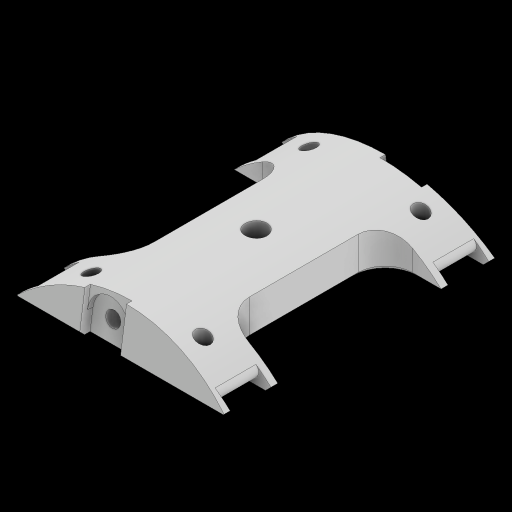
# Autodesk Inventor part: kozepso_csomopont
Saved by Autodesk Inventor 2023 (Build 270158000, 158)
## iProperties
Created: 2022-11-12
Part Number: kozepso_csomopont
Material: Generic
Document SubType Name: Modeling
Designer: gd1
Density: 1 g/cm^3
Appearance: Default
Author: gd1
Autodesk Inventor part; units mm, degrees
ref_plane "YZ Plane" through (0, 0, 0) normal (1, 0, 0) x (0, 1, 0)
ref_plane "XZ Plane" through (0, 0, 0) normal (0, 1, 0) x (-1, 0, 0)
ref_plane "XY Plane" through (0, 0, 0) normal (0, 0, 1) x (1, 0, 0)
sketch "Sketch1" plane through (0, 0, 0) normal (0, 1, 0) x (-1, 0, 0)
  line L0 (0, 90.017577) -> (-6, 90.017577)
  circle A0 centre (-3, 90.017577) radius 2.75
  circle A1 centre (-3, 90.017577) radius 7.5
  line L1 (17.5, 99.997436) -> (17.5, -0.002564)
  circle A2 centre (-3.002932, 9.980298) radius 7.5
  circle A3 centre (-3.002932, 9.980298) radius 2.75
  circle A4 centre (38.002932, 9.980298) radius 7.5
  circle A5 centre (38.002932, 9.980298) radius 2.75
  circle A6 centre (38, 90.017577) radius 7.5
  circle A7 centre (38, 90.017577) radius 2.75
  line L2 (38.002932, 9.980298) -> (-3.002932, 9.980298)
  line L3 (38, 90.017577) -> (-3, 90.017577)
  circle A8 centre (17.5, 49.997436) radius 10
  line L4 (35, 19.977295) -> (35, 80.017577)
  line L5 (0, 80.017577) -> (0, 19.977295)
  line L6 (-20.507033, 80.017577) -> (55.495326, 80.017577)
  line L7 (55.495326, 80.017577) -> (55.495326, 99.997436)
  line L8 (55.495326, 99.997436) -> (-20.507033, 99.997436)
  line L9 (-20.507033, 99.997436) -> (-20.507033, 80.017577)
  line L10 (-20.507033, 19.977295) -> (55.495326, 19.977295)
  line L11 (55.495326, 19.977295) -> (55.495326, -0.007838)
  line L12 (55.495326, -0.007838) -> (-20.507033, -0.007838)
  line L13 (-20.507033, -0.007838) -> (-20.507033, 19.977295)
  line L14 (55.495326, 97.517577) -> (-20.507033, 97.517577)
  line L15 (-20.507033, 82.517577) -> (55.495326, 82.517577)
  line L16 (55.495326, 17.480298) -> (-20.507033, 17.480298)
  line L17 (-20.507033, 2.480298) -> (55.495326, 2.480298)
  point P0 (-3, 82.517577)
  point P1 (0, 97.517577)
  point P2 (0, 0)
  point P3 (38.002932, 2.480298)
  point P4 (38.002932, 17.480298)
  point P5 (-3.002932, 2.480298)
  point P6 (-3.002932, 17.480298)
  point P7 (-3, 82.517577)
  point P8 (-3, 97.517577)
  point P9 (38, 82.517577)
  point P10 (38, 97.517577)
  point P11 (-3, 82.517577)
  dimension "d0" = 5.5
  dimension "d1" = 15
  dimension "d2" = 20
  dimension "d4" = 35
  constraints: 36 end point, 15 point on line, 9 centre point, 8 point on circle, 7 coincident, 6 perpendicular, 5 parallel, 4 horizontal, 4 symmetric about line, 1 midpoint, 4 other
  measures "d0" diameter of A0
  measures "d1" diameter of A1
  measures "d2" diameter of A8
  measures "d4" distance of L5.start L4.end
extrude "Extrusion1" add sketch "Sketch1" along normal blind 17 contours A0 L0 | L0 A0 | A1 | L3 L1 L15 A1 | A1 L14 L1 L3 | L14 L9 L8 L1 | A1 L15 L9 L14 | L15 L1 L6 L9 | L3 A6 L15 L1 | L1 L14 A6 L3 | L1 L8 L7 L14 | L15 L7 L6 L1 | A6 | L14 L7 L15 A6 | L6 L4 L10 L1 A8 | L1 A8 L10 L5 L6 | A8 L1 | L1 A8 | L10 L1 L16 L13 | L10 L11 L16 L1 | L16 A2 L17 L13 | L16 A4 L2 L1 | L1 L2 A2 L16 | L11 L17 A4 L16 | L17 L11 L12 L13 | A2 | L2 A4 L17 L1 | L1 L17 A2 L2 | A4 | A3 | A5 | A7
sketch "Sketch2" plane through (20.507033, 0, -0.007838) normal (0, 0, -1) x (-1, 0, 0)
  line L0 (76.002358, 0) -> (0, 0)
  line L1 (76.002358, 0) -> (76.002358, 17)
  line L2 (0, 0) -> (76.002358, 0)
  line L3 (76.002358, 0) -> (76.002358, 2)
  line L4 (76.002358, 2) -> (0, 2)
  line L5 (0, 2) -> (0, 0)
  circle A0 centre (38.001179, -38.636321) radius 55.636321
  line L6 (0, 17) -> (76.002358, 17)
  circle A1 centre (38.001179, -38.636321) radius 86.508977
  line L7 (38.001179, 2) -> (38.001179, 17)
  point P0 (20.507033, 0)
  point P1 (38.001179, 17)
  dimension "d7" = 2
  constraints: 10 end point, 2 horizontal, 2 midpoint, 2 parallel, 1 centre point, 1 coincident, 1 perpendicular, 1 point on line, 3 other
  measures "d7" distance of L3.end L2.end
extrude "Extrusion2" cut sketch "Sketch2" against normal blind 200 contours A0 L6 L1 | A1
fillet "Fillet2" radius 10 4 edges at (-35, 7.0871, 19.9773) (-35, 7.0871, 80.0176) (0, 7.089, 19.9773) (0, 7.089, 80.0176)
chamfer "Chamfer1" distance 2 angle 45 16 edges at (-35, 0, 49.9974) (-37.9289, 0, 77.0886) (-50.2477, 0, 80.0176) (-37.9289, 0, 22.9062) (-50.2477, 0, 19.9773) (-17.4941, 0, 99.9974) (-55.4953, 0, 90.0075) (-55.4953, 0, 9.9847) (-17.4941, 0, -0.0078) (20.507, 0, 9.9847) (15.2535, 0, 19.9773) (2.9289, 0, 22.9062) (0, 0, 49.9974) (2.9289, 0, 77.0886) (15.2535, 0, 80.0176) (20.507, 0, 90.0075)
ref_plane "Work Plane1" through (-17.5, 14.174145, 29.977295) normal (-1, 0, 0) x (0, 0, 1)
sketch "Sketch3" plane through (-17.5, 14.174145, 29.977295) normal (-1, 0, 0) x (0, 0, 1)
  line L0 (-29.985133, 2.825855) -> (-29.985133, -12.174145)
  line L1 (-29.985133, 2.825855) -> (70.014867, 2.825855)
  line L2 (-29.985133, 2.825855) -> (70.014867, 2.825855) construction
  line L3 (70.020141, 2.825855) -> (-29.985133, 2.825855)
  line L4 (20.017504, 2.825855) -> (20.017504, -14.174145)
  line L5 (40.040282, -14.174145) -> (0, -14.174145)
  line L6 (20.017504, 2.825855) -> (37.017504, 2.825855) construction
  line L7 (20.017504, -14.174145) -> (20.017504, 246.173645)
  line L8 (20.017504, -14.174145) -> (280.365294, -14.174145) construction
  line L9 (20.017504, -14.174145) -> (67.997363, -14.174145)
  line L10 (20.017504, 246.173645) -> (30.956214, 246.173645)
  line L11 (67.997363, -14.174145) -> (30.956214, 246.173645)
  line L12 (70.017504, -14.174145) -> (32.691804, 248.173645)
  line L13 (67.997363, -14.174145) -> (70.017504, -14.174145)
  line L14 (-27.962355, -14.174145) -> (9.078794, 246.173645)
  line L15 (-29.982496, -14.174145) -> (7.343204, 248.173645)
  line L16 (-27.962355, -14.174145) -> (-29.982496, -14.174145)
  line L17 (-37.762479, 9.08551) -> (76.654917, 9.08551)
  line L18 (76.654917, 9.08551) -> (76.654917, -19.464355)
  line L19 (76.654917, -19.464355) -> (-37.762479, -19.464355)
  line L20 (-37.762479, -19.464355) -> (-37.762479, 9.08551)
  line L21 (-27.985133, -14.174145) -> (20.017504, -14.174145)
  line L22 (7.343204, 248.173645) -> (32.691804, 248.173645)
  line L23 (9.078794, 246.173645) -> (20.017504, 246.173645)
  point P0 (-29.977295, -14.174145)
  point P1 (-26.673214, 9.08551)
  point P2 (66.708222, 9.08551)
  dimension "d18" = 100
  dimension "d20" = 90
  dimension "d21" = 260.34779
  dimension "d22" = 90
  dimension "d23" = 47.97986
  dimension "d24" = 10.93871
  dimension "d25" = 2
  constraints: 42 end point, 7 horizontal, 4 parallel, 4 symmetric about line, 3 equal length, 3 point on line, 1 midpoint, 1 perpendicular, 1 vertical
  measures "d18" distance of L0.start L1.end
  measures "d20" angle of L4 L6
  measures "d21" distance of L4.end L7.end
  measures "d22" angle of L8 L7
  measures "d23" distance of L4.end L9.end
  measures "d24" distance of L7.end L10.end
  measures "d25" distance between parallel lines of L11 L12
extrude "Extrusion3" cut sketch "Sketch3" along normal mid plane 200 contours L15 L16 L21 L5 L9 L13 L12 L17 L18 L19 L20
extrude "Extrusion4" cut sketch "Sketch1" along normal blind 2 contours A0 L0 | L0 A0 | A1 | A1 L15 L9 L14 | A6 | L14 L7 L15 A6 | L16 A2 L17 L13 | L11 L17 A4 L16 | A2 | A4 | A3 | A5 | A7
extrude "Extrusion5" cut sketch "Sketch1" along normal blind 3 contours A0 L0 | L0 A0 | A1 | A6 | A2 | A4 | A3 | A5 | A7
extrude "Extrusion6" cut sketch "Sketch1" along normal blind 15 contours A0 L0 | L0 A0 | A3 | A5 | A7
sketch "Sketch4" plane through (20.255615, 1.748582, 0.24358) normal (0, 0.1408571, -0.9900299) x (-1, 0, 0)
  ellipse E0 centre (37.749761, -40.791598) end of major axis (37.749761, 15.405007) minor radius 55.636321 (75.750941, 0.25395) -> (-0.251418, 0.25395) ccw
  line L0 (75.750941, 0.25395) -> (75.499523, 0)
  line L1 (-0.2365, 0.25395) -> (75.750941, 0.25395)
  line L2 (37.75722, 0.25395) -> (37.75722, 15.25395)
  line L3 (37.75722, 0.25395) -> (52.75722, 0.25395) construction
  line L4 (37.75722, 0.25395) -> (37.75722, -1.74605)
  line L5 (75.499523, 0) -> (0, 0)
  line L6 (37.75722, 0.25395) -> (39.75722, 0.25395) construction
  line L7 (37.75722, -1.484848) -> (22.75722, -1.484848)
  line L8 (22.75722, -1.74605) -> (22.75722, 13.25395)
  line L9 (22.75722, 13.515152) -> (37.75722, 13.515152)
  line L10 (37.75722, 13.515152) -> (37.75722, -1.484848)
  circle A0 centre (30.25722, 6.015152) radius 7.5
  circle A1 centre (30.25722, 6.015152) radius 2.75
  line L11 (22.75722, -1.484848) -> (22.75722, 18.515152)
  line L12 (22.75722, 18.515152) -> (37.75722, 18.515152)
  line L13 (37.75722, 18.515152) -> (37.75722, -1.484848)
  line L14 (1.748582, -1.484848) -> (73.750941, -1.484848)
  point P0 (20.255615, -1.765459)
  point P1 (37.75722, 15.25395)
  point P2 (22.75722, 13.25395)
  point P3 (30.25722, -1.74605)
  point P4 (30.25722, -1.484848)
  point P5 (30.25722, -1.484848)
  point P6 (37.75722, 6.015152)
  point P7 (22.75722, 6.015152)
  dimension "d35" = 15
  dimension "d36" = 90
  dimension "d37" = 2
  dimension "d38" = 90
  dimension "d39" = 15
  dimension "d40" = 15
  dimension "d41" = 5.5
  dimension "d42" = 20
  constraints: 24 end point, 4 horizontal, 4 perpendicular, 3 parallel, 2 centre point, 1 coincident, 1 midpoint, 1 point on line, 1 vertical, 1 other
  measures "d35" distance of L2.start L2.end
  measures "d36" angle of L3 L2
  measures "d37" distance of L4.end L2.start
  measures "d38" angle of L4 L6
  measures "d39" distance of L9.start L9.end
  measures "d40" distance of L8.start L8.end
  measures "d41" diameter of A1
  measures "d42" distance of L11.start L11.end
extrude "Extrusion10" cut sketch "Sketch4" against normal blind 4 contours L4 L5 A0 L1 | L1 A0 L2 | L4 L7 A0 L5 | A0 L5 L1 | L1 A0 | A0 L5 | A0 L5 L8 L1 | L1 L8 A0 | L7 L8 L5 A0 | A1
extrude "Extrusion11" cut sketch "Sketch4" against normal blind 2 fills toward (22.80722, 8.515152) open curves L11 L12 L13
extrude "Extrusion12" cut sketch "Sketch4" against normal blind 20 contours A1
sketch "Sketch5" plane through (-55.243908, 1.748582, 99.746019) normal (0, 0.1408571, 0.9900299) x (1, 0, 0)
  ellipse E0 centre (37.749761, -40.791598) end of major axis (37.749761, 15.405007) minor radius 55.636321 (75.750941, 0.25395) -> (-0.251418, 0.25395) ccw
  line L0 (75.750941, 0.25395) -> (75.499523, 0)
  line L1 (-0.2365, 0.25395) -> (75.750941, 0.25395)
  line L2 (37.75722, 0.25395) -> (37.75722, 15.25395)
  line L3 (37.75722, 0.25395) -> (52.75722, 0.25395) construction
  line L4 (37.75722, 0.25395) -> (37.75722, -1.74605)
  line L5 (75.499523, 0) -> (0, 0)
  line L6 (37.75722, 0.25395) -> (39.75722, 0.25395) construction
  line L7 (37.75722, -1.484848) -> (22.75722, -1.484848)
  line L8 (22.75722, -1.74605) -> (22.75722, 13.25395)
  line L9 (22.75722, 13.515152) -> (37.75722, 13.515152)
  line L10 (37.75722, 13.515152) -> (37.75722, -1.484848)
  circle A0 centre (30.25722, 6.015152) radius 7.5
  circle A1 centre (30.25722, 6.015152) radius 2.75
  line L11 (22.75722, -1.484848) -> (22.75722, 18.515152)
  line L12 (22.75722, 18.515152) -> (37.75722, 18.515152)
  line L13 (37.75722, 18.515152) -> (37.75722, -1.484848)
  line L14 (1.748582, -1.484848) -> (73.750941, -1.484848)
  point P0 (55.243908, 12.318791)
  point P1 (20.255615, -1.765459)
  point P2 (30.25722, -1.74605)
  point P3 (30.25722, -1.484848)
  point P4 (37.75722, 6.015152)
  point P5 (22.75722, 6.015152)
  point P6 (22.75722, -1.484848)
  point P7 (37.75722, -1.484848)
  point P8 (37.75722, 0.25395)
  dimension "d56" = 15
  dimension "d57" = 90
  dimension "d58" = 2
  dimension "d59" = 90
  dimension "d60" = 15
  dimension "d61" = 15
  dimension "d62" = 5.5
  dimension "d63" = 20
  constraints: 30 end point, 4 horizontal, 4 perpendicular, 3 parallel, 2 centre point, 1 coincident, 1 midpoint, 1 point on line, 1 vertical, 4 other
  measures "d56" distance of L4.start L2.end
  measures "d57" angle of L3 L2
  measures "d58" distance of L4.end L4.start
  measures "d59" angle of L4 L6
  measures "d60" distance of L9.start L10.start
  measures "d61" distance of L8.start L8.end
  measures "d62" diameter of A1
  measures "d63" distance of L11.start L12.start
extrude "Extrusion13" cut sketch "Sketch5" against normal blind 2 fills toward (22.80722, 8.515152) open curves L11 L12 L13
extrude "Extrusion14" cut sketch "Sketch5" against normal blind 4 contours L4 L5 A0 L1 | L1 A0 L2 | L4 L7 A0 L5 | A0 L5 L1 | L1 A0 | A0 L5 | A0 L5 L8 L1 | L1 L8 A0 | L7 L8 L5 A0 | A1
extrude "Extrusion15" cut sketch "Sketch5" against normal blind 20 contours A1
hole "Hole1" at (-17.5, 0, 49.997436) direction (0, 1, 0) diameter 8 depth 20
fillet "Fillet4" radius 2.5 4 edges at (20.507, 1.9999, 90.0176) (20.507, 1.9999, 9.9803) (-55.4953, 1.9999, 90.0176) (-55.4953, 1.9999, 9.9803)
body "Solid1"
